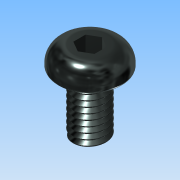
# Autodesk Inventor part: винт м4
Saved by Autodesk Inventor 2017 (Build 210142000, 142)
## iProperties
Part Number: винт м4
Material: Типовые
Document SubType Name: Modeling
Designer: Max
Mass: 0.063372 g
Surface Area: 2.34589 cm^2
Volume: 0.063372 cm^3
Density: 1 g/cm^3
Appearance: Оружейный металл — полированный
Author: Max
Autodesk Inventor part; units mm, degrees
ref_plane "YZ Plane" through (0, 0, 0) normal (1, 0, 0) x (0, 1, 0)
ref_plane "XZ Plane" through (0, 0, 0) normal (0, 1, 0) x (-1, 0, 0)
ref_plane "XY Plane" through (0, 0, 0) normal (0, 0, 1) x (1, 0, 0)
sketch "Эскиз1" plane through (0, 0, 0) normal (0, 0, 1) x (1, 0, 0)
  circle A0 centre (0, 0) radius 2.875
  line L0 (0, 1.0854) -> (0.94, 0.5427)
  line L1 (0.94, 0.5427) -> (0.94, -0.5427)
  line L2 (0.94, -0.5427) -> (0, -1.0854)
  line L3 (0, -1.0854) -> (-0.94, -0.5427)
  line L4 (-0.94, -0.5427) -> (-0.94, 0.5427)
  line L5 (-0.94, 0.5427) -> (0, 1.0854)
  circle A1 centre (0, 0) radius 1.5
  dimension "d0" = 5.75
  dimension "d1" = 1.88
  dimension "d2" = 3
  constraints: 12 end point, 3 coincident, 2 centre point, 13 other
  measures "d0" diameter of A0
  measures "d1" distance between parallel lines of L1 L4
  measures "d2" diameter of A1
extrude "Выдавливание1" add sketch "Эскиз1" against normal blind 5 contours L0 L1 L2 L3 L4 L5 | A1
extrude "Выдавливание2" add sketch "Эскиз1" along normal blind 1.88 contours A0 | A1
fillet "Сопряжение1" radius 1.4 1 edges at (-2.875, 0, 1.88)
fillet "Сопряжение2" radius 0.3 1 edges at (-2.875, 0, 0)
thread "Резьба2" size "M3x0.5" class "6g" standard "ANSI Metric M Profile" full length
sketch "Эскиз6" plane through (0, 0, -5) normal (1, 0, 0) x (0, 1, 0)
  line L0 (1.5, 0) -> (1.5, 5)
  line L1 (1.5, 5) -> (1.1293, 5)
  line L2 (1.1293, 5) -> (1.1293, 0)
  line L3 (1.1293, 0) -> (1.5, 0)
  line L4 (0, -2.0304) -> (0, 8.3651) projected
  constraints: 8 end point
revolve "Вращение3" cut sketch "Эскиз6" angle 360 about axis through (0, 0, -5) along (0, 0, 1)
sketch "Эскиз7" plane through (0, 0, -5) normal (1, 0, 0) x (0, 1, 0)
  line L0 (1.5, 0) -> (1.5, 5)
  line L1 (1.5, 5) -> (1.1293, 5)
  line L2 (1.1293, 5) -> (1.1293, 0)
  line L3 (1.1293, 0) -> (1.5, 0)
  line L4 (0, -2.0304) -> (0, 8.3651) projected
  constraints: 8 end point
revolve "Вращение4" add sketch "Эскиз7" angle 360 about axis through (0, 0, -5) along (0, 0, 1) separate body
sketch "Эскиз5" plane through (0, 0, -5) normal (-1, 0, 0) x (0, 0, 1)
  line L0 (-0.2918, -1.1547) -> (-0.2501, -1.1547) construction
  line L1 (0.0416, -1.4749) -> (-0.0001, -1.5549) construction
  line L2 (-0.5001, -1.5549) -> (-0.5418, -1.4749) construction
  line L3 (-0.2084, -1.1547) -> (-0.2501, -1.0747) construction
  line L4 (-0.2501, -1.0747) -> (-0.2918, -1.1547) construction
  line L5 (-0.5001, -1.5549) -> (-0.4584, -1.4749) construction
  line L6 (-0.2084, -1.1547) -> (-0.0418, -1.4749)
  line L7 (-0.5418, -1.4749) -> (-0.4584, -1.4749) construction
  arc A0 (-0.5418, -1.4749) -> (-0.5001, -1.5002) centre (-0.5001, -1.4532) ccw construction
  line L8 (0.0416, -1.4749) -> (-0.0418, -1.4749) construction
  line L9 (-0.5001, -1.5549) -> (-0.5001, -1.4749) construction
  line L10 (-0.0001, -1.5549) -> (-0.0001, -1.4749) construction
  line L11 (-0.2501, -1.0747) -> (-0.2501, -1.1294) construction
  line L12 (-0.5001, -1.5002) -> (-0.0001, -1.5002)
  arc A1 (-0.5001, -1.5002) -> (-0.4584, -1.4749) centre (-0.5001, -1.4532) ccw
  line L13 (-0.0418, -1.4749) -> (-0.0001, -1.5549) construction
  line L14 (-0.4584, -1.4749) -> (-0.2918, -1.1547)
  line L15 (-0.0001, -0.0002) -> (-0.0001, 0.0177)
  line L16 (-0.0001, 0.0177) -> (-0.0001, -0.0002)
  line L17 (-0.0001, -0.0002) -> (0.0334, -0.0002)
  arc A2 (-0.0418, -1.4749) -> (-0.0001, -1.5002) centre (-0.0001, -1.4532) ccw
  arc A3 (-0.0001, -1.5002) -> (0.0416, -1.4749) centre (-0.0001, -1.4532) ccw construction
  arc A4 (-0.2501, -1.1294) -> (-0.2918, -1.1547) centre (-0.2501, -1.1764) ccw
  arc A5 (-0.2084, -1.1547) -> (-0.2501, -1.1294) centre (-0.2501, -1.1764) ccw
  line L18 (-0.2501, -1.1294) -> (-0.2501, -1.1547) construction
  line L19 (-0.2501, -1.1547) -> (-0.2084, -1.1547) construction
  dimension "d32" = 55
  dimension "d33" = 0.08
  dimension "d34" = 0.08
  dimension "Эскиз5_ThreadOffset" = 0
  dimension "Эскиз5_MajorRadius" = 1.5
  dimension "d37" = 0.5
  dimension "Эскиз5_MinorRadius" = 1.1293
  constraints: 40 end point, 12 point on circle, 10 parallel, 8 tangent, 6 centre point, 6 collinear, 2 midpoint, 2 point on line, 1 horizontal, 1 perpendicular, 3 other
  measures "d32" angle of L6 L14
  measures "d33" distance of L3.end L0.end
  measures "d34" distance of L1.end L10.end
  measures "Эскиз5_ThreadOffset" distance between parallel lines of L15 L10
  measures "Эскиз5_MajorRadius" distance from line of L12 L15.start
  measures "d37" distance from line of L1.end L9
  measures "Эскиз5_MinorRadius" distance edge to line of A5 L17
coil "Пружина2" sketch "Эскиз5" operation cut axis through (0, 0, -5) along (0, 0, 1) pitch 0.5005 turns 11.988012 hand right bodies 2
equation "\"d32\" = d39"
equation "\"d33\" = 0.160083 * Эскиз5_Pitch"
equation "\"d34\" = 0.160083 * Эскиз5_Pitch"
equation "\"d37\" = Эскиз5_Pitch"
equation "\"d18\" = 55deg"
equation "\"Эскиз2_Pitch\" = 0.7"
equation "\"d39\" = 55deg"
equation "\"Эскиз5_Pitch\" = 0.5"
